Autodesk Inventor part; units mm, degrees
(part 2 of 2)
  spline S144 degree 2 poles (-13.6919, 16.6511) (-13.8375, 16.8177) (-14.1884, 16.8614) (-14.3941, 16.7606) knots 0 0 0 1 2 2 2
  spline S145 degree 2 poles (-14.3941, 16.7606) (-14.5313, 16.6935) (-14.921, 16.4885) (-15.0558, 16.4272) knots 0 0 0 1 2 2 2
  spline S146 degree 2 poles (-15.0558, 16.4272) (-15.3998, 16.2735) (-15.9448, 16.3885) (-16.1595, 16.6341) knots 0 0 0 1 2 2 2
  spline S147 degree 2 poles (-16.1595, 16.6341) (-16.2957, 16.79) (-16.431, 17.1991) (-16.4093, 17.4027) knots 0 0 0 1 2 2 2
  spline S148 degree 2 poles (-16.4093, 17.4027) (-16.3841, 17.6281) (-16.172, 18.032) (-15.9307, 18.2429) knots 0 0 0 1 2 2 2
  spline S149 degree 2 poles (-17.9083, 15.8045) (-17.901, 15.871) (-17.8822, 16.1006) (-17.8558, 16.192) knots 0 0 0 1 2 2 2
  spline S150 degree 2 poles (-17.8558, 16.192) (-17.8228, 16.3198) (-17.7227, 16.5246) (-17.5881, 16.6706) knots 0 0 0 1 2 2 2
  spline S151 degree 2 poles (-17.5881, 16.6706) (-17.4786, 16.7894) (-17.1909, 16.9215) (-17.0346, 16.9279) knots 0 0 0 1 2 2 2
  spline S152 degree 2 poles (-17.0346, 16.9279) (-16.8842, 16.9319) (-16.5641, 16.8104) (-16.4348, 16.6912) knots 0 0 0 1 2 2 2
  spline S153 degree 2 poles (-16.4348, 16.6912) (-16.2347, 16.5067) (-16.1068, 16.0763) (-16.1947, 15.8178) knots 0 0 0 1 2 2 2
  spline S154 degree 2 poles (-16.1947, 15.8178) (-16.2696, 15.5859) (-16.6209, 15.092) (-16.8428, 14.822) knots 0 0 0 1 2 2 2
  line L139 (-16.8428, 14.822) -> (-16.7802, 14.7644)
  spline S155 degree 2 poles (-16.7802, 14.7644) (-16.6676, 14.6605) (-16.4645, 14.6005) (-16.3672, 14.6265) knots 0 0 0 1 2 2 2
  spline S156 degree 2 poles (-16.3672, 14.6265) (-16.2699, 14.6526) (-16.0795, 14.8088) (-15.9911, 14.9047) knots 0 0 0 1 2 2 2
  spline S157 degree 2 poles (-15.9911, 14.9047) (-15.8872, 15.0173) (-15.6732, 15.3833) (-15.5975, 15.5951) knots 0 0 0 1 2 2 2
  line L140 (-15.5975, 15.5951) -> (-15.5802, 15.6139)
  line L141 (-15.5802, 15.6139) -> (-15.2487, 15.3082)
  spline S158 degree 2 poles (-15.2487, 15.3082) (-15.3063, 15.1955) (-15.5533, 14.8021) (-15.7052, 14.6373) knots 0 0 0 1 2 2 2
  spline S159 degree 2 poles (-15.7052, 14.6373) (-15.8898, 14.4372) (-16.2042, 14.2217) (-16.3855, 14.1882) knots 0 0 0 1 2 2 2
  spline S160 degree 2 poles (-16.3855, 14.1882) (-16.5628, 14.1549) (-16.9113, 14.2833) (-17.0927, 14.4506) knots 0 0 0 1 2 2 2
  line L142 (-17.0927, 14.4506) -> (-18.4126, 15.6676)
  line L143 (-18.4126, 15.6676) -> (-18.1127, 15.9929)
  line L144 (-18.1127, 15.9929) -> (-17.9083, 15.8045)
  line L145 (-17.6372, 15.5546) -> (-17.1013, 15.0604)
  spline S161 degree 2 poles (-17.1013, 15.0604) (-17.0041, 15.1868) (-16.7146, 15.5719) (-16.6461, 15.7132) knots 0 0 0 1 2 2 2
  spline S162 degree 2 poles (-16.6461, 15.7132) (-16.5665, 15.879) (-16.5755, 16.1998) (-16.7214, 16.3344) knots 0 0 0 1 2 2 2
  spline S163 degree 2 poles (-16.7214, 16.3344) (-16.8883, 16.4882) (-17.2302, 16.4563) (-17.3955, 16.2769) knots 0 0 0 1 2 2 2
  spline S164 degree 2 poles (-17.3955, 16.2769) (-17.5359, 16.1247) (-17.6353, 15.7534) (-17.6372, 15.5546) knots 0 0 0 1 2 2 2
  line L146 (-19.0748, 14.8248) -> (-18.8001, 15.1716)
  line L147 (-18.8001, 15.1716) -> (-15.934, 12.9018)
  line L148 (-15.934, 12.9018) -> (-16.2088, 12.5549)
  line L149 (-16.2088, 12.5549) -> (-19.0748, 14.8248)
  line L150 (-20.4524, 12.8928) -> (-19.3588, 14.4815)
  line L151 (-19.3588, 14.4815) -> (-19.0878, 14.295)
  line L152 (-19.0878, 14.295) -> (-18.2728, 12.0674)
  line L153 (-18.2728, 12.0674) -> (-17.5266, 13.1515)
  line L154 (-17.5266, 13.1515) -> (-17.2275, 12.9457)
  line L155 (-17.2275, 12.9457) -> (-18.2744, 11.4247)
  line L156 (-18.2744, 11.4247) -> (-18.5338, 11.6032)
  line L157 (-18.5338, 11.6032) -> (-19.3503, 13.8386)
  line L158 (-19.3503, 13.8386) -> (-20.1463, 12.6821)
  line L159 (-20.1463, 12.6821) -> (-20.4524, 12.8928)
  spline S165 degree 2 poles (-20.5457, 9.9599) (-21.1096, 10.2705) (-21.4967, 11.1962) (-21.2695, 11.6086) knots 0 0 0 1 2 2 2
  spline S166 degree 2 poles (-21.2695, 11.6086) (-21.1668, 11.7949) (-20.9284, 12.0101) (-20.7778, 12.0954) knots 0 0 0 1 2 2 2
  line L160 (-20.7778, 12.0954) -> (-20.8709, 12.1791)
  line L161 (-20.8709, 12.1791) -> (-20.6711, 12.5418)
  line L162 (-20.6711, 12.5418) -> (-17.4689, 10.7776)
  line L163 (-17.4689, 10.7776) -> (-17.6824, 10.39)
  line L164 (-17.6824, 10.39) -> (-18.8252, 11.0196)
  spline S167 degree 2 poles (-18.8252, 11.0196) (-18.7743, 10.8005) (-18.7879, 10.3644) (-18.907, 10.1483) knots 0 0 0 1 2 2 2
  spline S168 degree 2 poles (-18.907, 10.1483) (-19.1219, 9.7582) (-19.9918, 9.6546) (-20.5457, 9.9599) knots 0 0 0 1 2 2 2
  spline S169 degree 2 poles (-20.3552, 10.3762) (-19.9428, 10.149) (-19.3773, 10.1645) (-19.224, 10.4427) knots 0 0 0 1 2 2 2
  spline S170 degree 2 poles (-19.224, 10.4427) (-19.1378, 10.5993) (-19.1089, 11.0043) (-19.1506, 11.1989) knots 0 0 0 1 2 2 2
  line L165 (-19.1506, 11.1989) -> (-20.4697, 11.9257)
  spline S171 degree 2 poles (-20.4697, 11.9257) (-20.6225, 11.8189) (-20.8067, 11.6256) (-20.8806, 11.4915) knots 0 0 0 1 2 2 2
  spline S172 degree 2 poles (-20.8806, 11.4915) (-21.0435, 11.1959) (-20.8098, 10.6267) (-20.3552, 10.3762) knots 0 0 0 1 2 2 2
  line L166 (-22.7058, 8.3102) -> (-22.5363, 8.7189)
  line L167 (-22.5363, 8.7189) -> (-22.2691, 8.6081)
  spline S173 degree 2 poles (-22.2691, 8.6081) (-22.3559, 8.8652) (-22.3861, 9.2738) (-22.2992, 9.4834) knots 0 0 0 1 2 2 2
  spline S174 degree 2 poles (-22.2992, 9.4834) (-22.234, 9.6406) (-22.0129, 9.8775) (-21.8579, 9.9329) knots 0 0 0 1 2 2 2
  spline S175 degree 2 poles (-21.8579, 9.9329) (-21.7018, 9.991) (-21.3108, 9.964) (-21.0645, 9.8618) knots 0 0 0 1 2 2 2
  line L168 (-21.0645, 9.8618) -> (-19.4899, 9.2089)
  line L169 (-19.4899, 9.2089) -> (-19.6594, 8.8002)
  line L170 (-19.6594, 8.8002) -> (-21.0427, 9.3738)
  spline S176 degree 2 poles (-21.0427, 9.3738) (-21.2366, 9.4542) (-21.5027, 9.5308) (-21.6176, 9.5201) knots 0 0 0 1 2 2 2
  spline S177 degree 2 poles (-21.6176, 9.5201) (-21.7326, 9.5094) (-21.8897, 9.375) (-21.956, 9.2152) knots 0 0 0 1 2 2 2
  spline S178 degree 2 poles (-21.956, 9.2152) (-22.0179, 9.0658) (-21.9877, 8.6572) (-21.9233, 8.4647) knots 0 0 0 1 2 2 2
  line L171 (-21.9233, 8.4647) -> (-20.1102, 7.7129)
  line L172 (-20.1102, 7.7129) -> (-20.2797, 7.3042)
  line L173 (-20.2797, 7.3042) -> (-22.7058, 8.3102)
  line L174 (-21.2617, 5.7315) -> (-21.255, 5.7532)
  spline S179 degree 2 poles (-21.255, 5.7532) (-21.2263, 5.7977) (-21.188, 5.9017) (-21.1652, 5.9748) knots 0 0 0 1 2 2 2
  spline S180 degree 2 poles (-21.1652, 5.9748) (-21.1121, 6.1454) (-21.1566, 6.5276) (-21.2556, 6.7248) knots 0 0 0 1 2 2 2
  line L175 (-21.2556, 6.7248) -> (-23.0349, 7.2785)
  line L176 (-23.0349, 7.2785) -> (-22.9034, 7.701)
  line L177 (-22.9034, 7.701) -> (-20.3956, 6.9205)
  line L178 (-20.3956, 6.9205) -> (-20.5271, 6.498)
  line L179 (-20.5271, 6.498) -> (-20.9008, 6.6143)
  spline S181 degree 2 poles (-20.9008, 6.6143) (-20.7666, 6.3201) (-20.7058, 5.9239) (-20.7563, 5.7614) knots 0 0 0 1 2 2 2
  spline S182 degree 2 poles (-20.7563, 5.7614) (-20.7766, 5.6964) (-20.8022, 5.6331) (-20.823, 5.595) knots 0 0 0 1 2 2 2
  line L180 (-20.823, 5.595) -> (-21.2617, 5.7315)
  spline S183 degree 2 poles (-23.8414, 6.038) (-23.8703, 5.9978) (-23.9675, 5.8416) (-24.0156, 5.7388) knots 0 0 0 1 2 2 2
  spline S184 degree 2 poles (-24.0156, 5.7388) (-24.0716, 5.6261) (-24.151, 5.4313) (-24.1765, 5.312) knots 0 0 0 1 2 2 2
  spline S185 degree 2 poles (-24.1765, 5.312) (-24.2192, 5.1124) (-24.1732, 4.8124) (-24.0955, 4.7146) knots 0 0 0 1 2 2 2
  spline S186 degree 2 poles (-24.0955, 4.7146) (-24.0172, 4.6196) (-23.7828, 4.5085) (-23.6248, 4.4747) knots 0 0 0 1 2 2 2
  line L181 (-23.6248, 4.4747) -> (-23.4001, 4.4266)
  spline S187 degree 2 poles (-23.4001, 4.4266) (-23.5153, 4.634) (-23.5877, 5.0004) (-23.5337, 5.2528) knots 0 0 0 1 2 2 2
  spline S188 degree 2 poles (-23.5337, 5.2528) (-23.4399, 5.691) (-22.6772, 6.0702) (-22.0642, 5.9391) knots 0 0 0 1 2 2 2
  spline S189 degree 2 poles (-22.0642, 5.9391) (-21.7453, 5.8708) (-21.2901, 5.5849) (-21.1475, 5.3978) knots 0 0 0 1 2 2 2
  spline S190 degree 2 poles (-21.1475, 5.3978) (-21.0147, 5.2185) (-20.9193, 4.7833) (-20.9644, 4.5726) knots 0 0 0 1 2 2 2
  spline S191 degree 2 poles (-20.9644, 4.5726) (-21.0071, 4.3729) (-21.1637, 4.1018) (-21.2811, 3.9732) knots 0 0 0 1 2 2 2
  line L182 (-21.2811, 3.9732) -> (-21.1783, 3.9251)
  line L183 (-21.1783, 3.9251) -> (-21.2655, 3.5174)
  line L184 (-21.2655, 3.5174) -> (-23.5398, 4.004)
  spline S192 degree 2 poles (-23.5398, 4.004) (-24.1944, 4.1441) (-24.6829, 4.8432) (-24.5577, 5.4284) knots 0 0 0 1 2 2 2
  spline S193 degree 2 poles (-24.5577, 5.4284) (-24.5173, 5.617) (-24.3721, 5.9978) (-24.2859, 6.1563) knots 0 0 0 1 2 2 2
  line L185 (-24.2859, 6.1563) -> (-23.8366, 6.0602)
  line L186 (-23.8366, 6.0602) -> (-23.8414, 6.038)
  line L187 (-23.0451, 4.3506) -> (-21.6334, 4.0486)
  spline S194 degree 2 poles (-21.6334, 4.0486) (-21.5213, 4.1928) (-21.3966, 4.4504) (-21.3675, 4.5863) knots 0 0 0 1 2 2 2
  spline S195 degree 2 poles (-21.3675, 4.5863) (-21.2975, 4.9136) (-21.6994, 5.394) (-22.1514, 5.4908) knots 0 0 0 1 2 2 2
  spline S196 degree 2 poles (-22.1514, 5.4908) (-22.5786, 5.5822) (-23.0862, 5.392) (-23.1551, 5.0703) knots 0 0 0 1 2 2 2
  spline S197 degree 2 poles (-23.1551, 5.0703) (-23.1913, 4.9011) (-23.1341, 4.5176) (-23.0451, 4.3506) knots 0 0 0 1 2 2 2
  constraints: 1 centre point, 1 coincident, 1 other
extrude "Extrusion3" add sketch "Skizze3" along normal blind 1 contours S0 S1 L0 L1 L2 L3 L4 S2 S3 | S8 S9 S10 S11 S12 S13 L8 S14 S15 S16 L9 L10 S17 S18 S19 L11 L12 L13 | L15 S24 S25 L16 L17 L18 L19 L20 S26 S27 L21 | L22 L23 L24 L25 | L26 L27 L28 L29 | S28 L30 L31 S29 S30 S31 S32 S33 S34 S35 S36 S37 L32 L33 S38 S39 S40 S41 S42 S43 S44 | L34 L35 L36 L37 L38 L39 | S45 S46 S47 S48 | L40 L41 S53 S54 S55 S56 S57 S58 S59 L42 L43 L44 | L46 S64 S65 L47 L48 L49 L50 L51 S66 S67 L52 | S68 S69 S70 S71 | L53 L54 S76 S77 S78 L55 L56 L57 L58 L59 S79 S80 L60 | S81 S82 L61 L62 L63 S83 S84 S85 S86 L64 L65 L66 S87 S88 | L67 L68 S89 S90 S91 L69 L70 L71 L72 L73 S92 S93 L74 | L75 L76 L77 L78 | L79 L80 L81 L82 | L83 L84 L85 L86 L87 L88 L89 | S94 S95 S96 S97 L90 L91 S98 S99 S100 L92 L93 S101 S102 | L95 S107 S108 L96 L97 L98 L99 L100 S109 S110 L101 | S111 L102 L103 S112 S113 S114 S115 S116 S117 S118 S119 S120 L104 L105 S121 S122 S123 S124 S125 S126 S127 | L106 L107 L108 L109 | L110 L111 L112 L113 | S128 L114 L115 L116 L117 L118 L119 L120 L121 L122 L131 L130 L123 L124 S129 S130 S131 L125 L126 S132 | L130 L131 L122 L123 | L123 L122 L131 L132 L133 L134 L127 L128 L129 L130 | S133 L135 L136 S134 S135 S136 S137 S138 S139 S140 S141 L137 L138 S142 S143 S144 S145 S146 S147 S148 | S149 S150 S151 S152 S153 S154 L139 S155 S156 S157 L140 L141 S158 S159 S160 L142 L143 L144 | L146 L147 L148 L149 | L150 L151 L152 L153 L154 L155 L156 L157 L158 L159 | S165 S166 L160 L161 L162 L163 L164 S167 S168 | L166 L167 S173 S174 S175 L168 L169 L170 S176 S177 S178 L171 L172 L173 | L174 S179 S180 L175 L176 L177 L178 L179 S181 S182 L180 | S183 S184 S185 S186 L181 S187 S188 S189 S190 S191 L182 L183 L184 S192 S193 L185 L186
